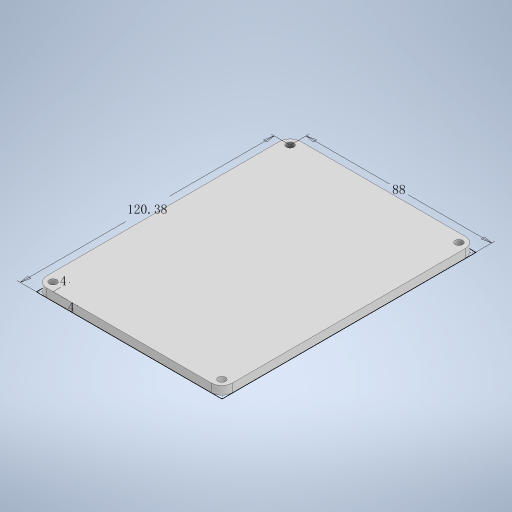
# Autodesk Inventor part: PrismGCUpNew
Saved by Autodesk Inventor 2024 (Build 280153000, 153)
## iProperties
Created: 2023-08-09
Part Number: PrismGCUpNew
Material: 常规
Document SubType Name: Modeling
Designer: liyuxuan
Density: 1 g/cm^3
Appearance: 默认
Author: liyuxuan
Autodesk Inventor part; units mm, degrees
ref_plane "YZ Plane" through (0, 0, 0) normal (1, 0, 0) x (0, 1, 0)
ref_plane "XZ Plane" through (0, 0, 0) normal (0, 1, 0) x (-1, 0, 0)
ref_plane "XY Plane" through (0, 0, 0) normal (0, 0, 1) x (1, 0, 0)
sketch "草图1" plane through (0, 0, 0) normal (0, 1, 0) x (-1, 0, 0)
  line L0 (-44, 60.19) -> (44, 60.19)
  line L1 (44, 60.19) -> (44, -60.19)
  line L2 (44, -60.19) -> (-44, -60.19)
  line L3 (-44, -60.19) -> (-44, 60.19)
  line L4 (-44, 60.19) -> (44, -60.19) construction
  line L5 (44, 60.19) -> (-44, -60.19) construction
  line L6 (0, 60.19) -> (0, -60.19)
  line L7 (44, 0) -> (-44, 0)
  point P0 (0, 0)
  point P1 (40, 56.19)
  point P2 (40, -56.19)
  point P3 (-40, 56.19)
  point P4 (-40, -56.19)
  dimension "d0" = 88
  dimension "d1" = 120.38
  dimension "d2" = 4
  dimension "d3" = 4
  constraints: 16 end point, 6 midpoint, 3 symmetric about line, 2 parallel, 1 horizontal, 1 perpendicular
  measures "d0" distance of L1.end L2.end
  measures "d1" distance of L0.end L1.end
  measures "d2" distance from line of L0 point (40, 56.19)
  measures "d3" distance from line of L1 point (40, 56.19)
extrude "拉伸1" add sketch "草图1" along normal blind 4
hole "孔1" at (-40, 0, 56.19) at (-40, 0, -56.19) at (40, 0, 56.19) at (40, 0, -56.19) direction (0, 1, 0) diameter 3.5 end through all
fillet "面圆角1" radius 5 1 edges at (44, 2, 60.19)
fillet "面圆角2" radius 5 1 edges at (-44, 2, 60.19)
fillet "面圆角3" radius 5 1 edges at (44, 2, -60.19)
fillet "面圆角4" radius 5 1 edges at (-44, 2, -60.19)
